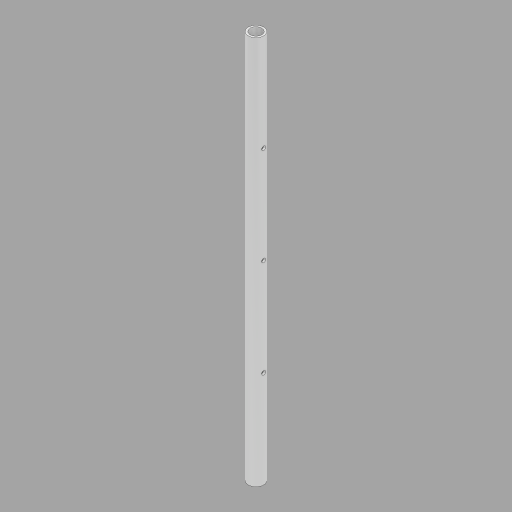
# Autodesk Inventor part: InsertTube4OD0.5W100L
Saved by Autodesk Inventor 2024 (Build 280153020, 153B)
## iProperties
Created: 2023-09-24
Part Number: InsertTube4OD0.5W100L
Material: Stainless Steel AISI 304
Document SubType Name: Modeling
Designer: schanen
Density: 8 g/cm^3
Appearance: Chrome - Satin
Author: schanen
Autodesk Inventor part; units mm, degrees
ref_plane "XZ Plane" through (0, 0, 0) normal (0, 1, 0) x (-1, 0, 0)
sketch "Sketch1" plane through (0, 0, 0) normal (0, 0, 1) x (1, 0, 0)
  line L0 (-1.5, 0) -> (-2, 0)
  line L1 (-2, 0) -> (-2, 100)
  line L2 (-2, 100) -> (-1.5, 100)
  line L3 (-1.5, 100) -> (-1.5, 0)
  line L4 (0, -20) -> (0, 120) projected
  point P0 (0, 0)
  dimension "d0" = 2
  dimension "d1" = 0.5
  dimension "d2" = 100
  constraints: 8 end point, 2 parallel, 1 horizontal, 1 perpendicular
  measures "d0" distance from line of point (0, 0) L1
  measures "d1" distance between parallel lines of L1 L3
  measures "d2" distance of L0.end L1.end
revolve "Revolution1" add sketch "Sketch1" angle 360 about axis through (0, -10, 0) along (0, 1, 0)
ref_plane "Work Plane1" through (0, 50, 0) normal (0, 1, 0) x (1, 0, 0)
ref_plane "Work Plane2" through (0, 0, 0) normal (1, 0, 0) x (0, 1, 0)
sketch "Sketch2" plane through (0, 0, 0) normal (1, 0, 0) x (0, 1, 0)
  line L0 (50, 2.8) -> (50, -2.8) projected
  line L1 (-1, 0) -> (6, 0) projected
  point P0 (0, 0)
  point P1 (50, 0)
  constraints: 1 midpoint, 1 point on line
hole "Hole1" at (0, 50, 0) direction (-1, 0, 0) diameter 1 end through all both
pattern_linear "Rectangular Pattern1" count 3 spacing 25 along (0, 1, 0) of "Hole1" first direction both ways yes
body "Solid1"
